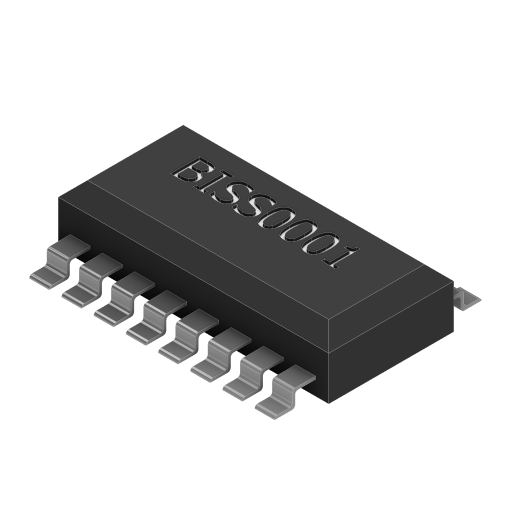
# Autodesk Inventor part: BISS0001 Chip
Saved by Autodesk Inventor 2024 (Build 280153000, 153)
## iProperties
Created: 2024-09-23
Part Number: BISS0001 Chip
Material: Generic
Document SubType Name: Modeling
Designer: Laith Al-Sadi
Density: 1 g/cm^3
Appearance: Rubber - Black
Author: Laith Al-Sadi
Autodesk Inventor part; units mm, degrees
ref_plane "YZ Plane" through (0, 0, 0) normal (1, 0, 0) x (0, 1, 0)
ref_plane "XZ Plane" through (0, 0, 0) normal (0, 1, 0) x (-1, 0, 0)
sketch "Sketch1" plane through (0, 0, 0) normal (0, 1, 0) x (-1, 0, 0)
  line L0 (4.62, 2.135) -> (-4.62, 2.135)
  line L1 (-4.62, 2.135) -> (-4.62, -2.135)
  line L2 (-4.62, -2.135) -> (4.62, -2.135)
  line L3 (4.62, -2.135) -> (4.62, 2.135)
  line L4 (4.62, 2.135) -> (-4.62, -2.135) construction
  line L5 (-4.62, 2.135) -> (4.62, -2.135) construction
  point P0 (0, 0)
  dimension "d0" = 9.24
  dimension "d1" = 4.27
  constraints: 12 end point, 2 midpoint, 2 parallel, 1 horizontal, 1 perpendicular
  measures "d0" distance of L1.end L2.end
  measures "d1" distance of L2.end L0.start
extrude "Extrusion1" add sketch "Sketch1" along normal blind 2
chamfer "Chamfer1" distance 0.5 angle 45 4 edges at (0, 2, 2.135) (-4.62, 2, 0) (0, 2, -2.135) (4.62, 2, 0)
sketch "Sketch2" plane through (0, 2, 0) normal (0, 1, 0) x (1, 0, 0)
  line L0 (-3, 1) -> (3, 1) construction
  line L1 (3, 1) -> (3, -1) construction
  line L2 (3, -1) -> (-3, -1) construction
  line L3 (-3, -1) -> (-3, 1) construction
  spline S0 degree 2 poles (-2.2204, 0.2869) (-2.2204, 0.2123) (-2.2771, 0.0981) (-2.3241, 0.0608) knots 0 0 0 1 2 2 2
  spline S1 degree 2 poles (-2.3241, 0.0608) (-2.3809, 0.017) (-2.5097, -0.0203) (-2.6118, -0.0203) knots 0 0 0 1 2 2 2
  line L4 (-2.6118, -0.0203) -> (-2.8987, -0.0203)
  line L5 (-2.8987, -0.0203) -> (-2.8987, 0.9797)
  line L6 (-2.8987, 0.9797) -> (-2.6337, 0.9797)
  spline S2 degree 2 poles (-2.6337, 0.9797) (-2.5267, 0.9797) (-2.4198, 0.966) (-2.3712, 0.9392) knots 0 0 0 1 2 2 2
  spline S3 degree 2 poles (-2.3712, 0.9392) (-2.3169, 0.9109) (-2.2674, 0.8177) (-2.2674, 0.7545) knots 0 0 0 1 2 2 2
  spline S4 degree 2 poles (-2.2674, 0.7545) (-2.2674, 0.684) (-2.342, 0.5721) (-2.4076, 0.5405) knots 0 0 0 1 2 2 2
  line L7 (-2.4076, 0.5405) -> (-2.4076, 0.5357)
  spline S5 degree 2 poles (-2.4076, 0.5357) (-2.3185, 0.5113) (-2.2204, 0.3825) (-2.2204, 0.2869) knots 0 0 0 1 2 2 2
  spline S6 degree 2 poles (-2.359, 0.2812) (-2.359, 0.3379) (-2.3914, 0.4109) (-2.44, 0.4368) knots 0 0 0 1 2 2 2
  spline S7 degree 2 poles (-2.44, 0.4368) (-2.4716, 0.453) (-2.5462, 0.4627) (-2.6151, 0.4627) knots 0 0 0 1 2 2 2
  line L8 (-2.6151, 0.4627) -> (-2.7658, 0.4627)
  line L9 (-2.7658, 0.4627) -> (-2.7658, 0.0932)
  line L10 (-2.7658, 0.0932) -> (-2.658, 0.0932)
  spline S8 degree 2 poles (-2.658, 0.0932) (-2.5705, 0.0932) (-2.47, 0.1094) (-2.4311, 0.1353) knots 0 0 0 1 2 2 2
  spline S9 degree 2 poles (-2.4311, 0.1353) (-2.3938, 0.1621) (-2.359, 0.2285) (-2.359, 0.2812) knots 0 0 0 1 2 2 2
  spline S10 degree 2 poles (-2.406, 0.7358) (-2.406, 0.7715) (-2.4303, 0.825) (-2.4571, 0.8404) knots 0 0 0 1 2 2 2
  spline S11 degree 2 poles (-2.4571, 0.8404) (-2.4895, 0.8582) (-2.5681, 0.8663) (-2.6386, 0.8663) knots 0 0 0 1 2 2 2
  line L11 (-2.6386, 0.8663) -> (-2.7658, 0.8663)
  line L12 (-2.7658, 0.8663) -> (-2.7658, 0.5737)
  line L13 (-2.7658, 0.5737) -> (-2.6151, 0.5737)
  spline S12 degree 2 poles (-2.6151, 0.5737) (-2.5527, 0.5737) (-2.4935, 0.5867) (-2.4619, 0.607) knots 0 0 0 1 2 2 2
  spline S13 degree 2 poles (-2.4619, 0.607) (-2.4311, 0.6264) (-2.406, 0.6888) (-2.406, 0.7358) knots 0 0 0 1 2 2 2
  line L14 (-1.7399, -0.0203) -> (-2.1272, -0.0203)
  line L15 (-2.1272, -0.0203) -> (-2.1272, 0.0818)
  line L16 (-2.1272, 0.0818) -> (-2, 0.0818)
  line L17 (-2, 0.0818) -> (-2, 0.8776)
  line L18 (-2, 0.8776) -> (-2.1272, 0.8776)
  line L19 (-2.1272, 0.8776) -> (-2.1272, 0.9797)
  line L20 (-2.1272, 0.9797) -> (-1.7399, 0.9797)
  line L21 (-1.7399, 0.9797) -> (-1.7399, 0.8776)
  line L22 (-1.7399, 0.8776) -> (-1.8671, 0.8776)
  line L23 (-1.8671, 0.8776) -> (-1.8671, 0.0818)
  line L24 (-1.8671, 0.0818) -> (-1.7399, 0.0818)
  line L25 (-1.7399, 0.0818) -> (-1.7399, -0.0203)
  spline S14 degree 2 poles (-1.2966, -0.0381) (-1.4052, -0.0381) (-1.5575, 0.0073) (-1.6248, 0.0397) knots 0 0 0 1 2 2 2
  line L26 (-1.6248, 0.0397) -> (-1.6248, 0.2066)
  line L27 (-1.6248, 0.2066) -> (-1.6151, 0.2066)
  spline S15 degree 2 poles (-1.6151, 0.2066) (-1.5494, 0.1451) (-1.3833, 0.077) (-1.3063, 0.077) knots 0 0 0 1 2 2 2
  spline S16 degree 2 poles (-1.3063, 0.077) (-1.1961, 0.077) (-1.0835, 0.1686) (-1.0835, 0.2439) knots 0 0 0 1 2 2 2
  spline S17 degree 2 poles (-1.0835, 0.2439) (-1.0835, 0.3039) (-1.1426, 0.3784) (-1.2066, 0.3971) knots 0 0 0 1 2 2 2
  spline S18 degree 2 poles (-1.2066, 0.3971) (-1.2528, 0.41) (-1.3298, 0.4279) (-1.3874, 0.4425) knots 0 0 0 1 2 2 2
  spline S19 degree 2 poles (-1.3874, 0.4425) (-1.4392, 0.4562) (-1.5211, 0.4976) (-1.5527, 0.5308) knots 0 0 0 1 2 2 2
  spline S20 degree 2 poles (-1.5527, 0.5308) (-1.5835, 0.564) (-1.6175, 0.6532) (-1.6175, 0.7115) knots 0 0 0 1 2 2 2
  spline S21 degree 2 poles (-1.6175, 0.7115) (-1.6175, 0.8331) (-1.4279, 0.9976) (-1.2812, 0.9976) knots 0 0 0 1 2 2 2
  spline S22 degree 2 poles (-1.2812, 0.9976) (-1.1969, 0.9976) (-1.0478, 0.9643) (-0.9838, 0.9327) knots 0 0 0 1 2 2 2
  line L28 (-0.9838, 0.9327) -> (-0.9838, 0.7739)
  line L29 (-0.9838, 0.7739) -> (-0.9935, 0.7739)
  spline S23 degree 2 poles (-0.9935, 0.7739) (-1.0413, 0.8177) (-1.1904, 0.8825) (-1.2723, 0.8825) knots 0 0 0 1 2 2 2
  spline S24 degree 2 poles (-1.2723, 0.8825) (-1.3647, 0.8825) (-1.4789, 0.7958) (-1.4789, 0.7253) knots 0 0 0 1 2 2 2
  spline S25 degree 2 poles (-1.4789, 0.7253) (-1.4789, 0.6621) (-1.4117, 0.5867) (-1.3485, 0.5697) knots 0 0 0 1 2 2 2
  spline S26 degree 2 poles (-1.3485, 0.5697) (-1.3063, 0.5583) (-1.184, 0.5292) (-1.1434, 0.517) knots 0 0 0 1 2 2 2
  spline S27 degree 2 poles (-1.1434, 0.517) (-1.0405, 0.4854) (-0.9449, 0.3582) (-0.9449, 0.265) knots 0 0 0 1 2 2 2
  spline S28 degree 2 poles (-0.9449, 0.265) (-0.9449, 0.2058) (-0.9927, 0.0924) (-1.0357, 0.0527) knots 0 0 0 1 2 2 2
  spline S29 degree 2 poles (-1.0357, 0.0527) (-1.0835, 0.0089) (-1.205, -0.0381) (-1.2966, -0.0381) knots 0 0 0 1 2 2 2
  spline S30 degree 2 poles (-0.5308, -0.0381) (-0.6394, -0.0381) (-0.7917, 0.0073) (-0.859, 0.0397) knots 0 0 0 1 2 2 2
  line L30 (-0.859, 0.0397) -> (-0.859, 0.2066)
  line L31 (-0.859, 0.2066) -> (-0.8493, 0.2066)
  spline S31 degree 2 poles (-0.8493, 0.2066) (-0.7836, 0.1451) (-0.6175, 0.077) (-0.5405, 0.077) knots 0 0 0 1 2 2 2
  spline S32 degree 2 poles (-0.5405, 0.077) (-0.4303, 0.077) (-0.3177, 0.1686) (-0.3177, 0.2439) knots 0 0 0 1 2 2 2
  spline S33 degree 2 poles (-0.3177, 0.2439) (-0.3177, 0.3039) (-0.3768, 0.3784) (-0.4408, 0.3971) knots 0 0 0 1 2 2 2
  spline S34 degree 2 poles (-0.4408, 0.3971) (-0.487, 0.41) (-0.564, 0.4279) (-0.6216, 0.4425) knots 0 0 0 1 2 2 2
  spline S35 degree 2 poles (-0.6216, 0.4425) (-0.6734, 0.4562) (-0.7553, 0.4976) (-0.7869, 0.5308) knots 0 0 0 1 2 2 2
  spline S36 degree 2 poles (-0.7869, 0.5308) (-0.8177, 0.564) (-0.8517, 0.6532) (-0.8517, 0.7115) knots 0 0 0 1 2 2 2
  spline S37 degree 2 poles (-0.8517, 0.7115) (-0.8517, 0.8331) (-0.6621, 0.9976) (-0.5154, 0.9976) knots 0 0 0 1 2 2 2
  spline S38 degree 2 poles (-0.5154, 0.9976) (-0.4311, 0.9976) (-0.282, 0.9643) (-0.218, 0.9327) knots 0 0 0 1 2 2 2
  line L32 (-0.218, 0.9327) -> (-0.218, 0.7739)
  line L33 (-0.218, 0.7739) -> (-0.2277, 0.7739)
  spline S39 degree 2 poles (-0.2277, 0.7739) (-0.2755, 0.8177) (-0.4246, 0.8825) (-0.5065, 0.8825) knots 0 0 0 1 2 2 2
  spline S40 degree 2 poles (-0.5065, 0.8825) (-0.5989, 0.8825) (-0.7131, 0.7958) (-0.7131, 0.7253) knots 0 0 0 1 2 2 2
  spline S41 degree 2 poles (-0.7131, 0.7253) (-0.7131, 0.6621) (-0.6459, 0.5867) (-0.5827, 0.5697) knots 0 0 0 1 2 2 2
  spline S42 degree 2 poles (-0.5827, 0.5697) (-0.5405, 0.5583) (-0.4182, 0.5292) (-0.3776, 0.517) knots 0 0 0 1 2 2 2
  spline S43 degree 2 poles (-0.3776, 0.517) (-0.2747, 0.4854) (-0.1791, 0.3582) (-0.1791, 0.265) knots 0 0 0 1 2 2 2
  spline S44 degree 2 poles (-0.1791, 0.265) (-0.1791, 0.2058) (-0.2269, 0.0924) (-0.2699, 0.0527) knots 0 0 0 1 2 2 2
  spline S45 degree 2 poles (-0.2699, 0.0527) (-0.3177, 0.0089) (-0.4392, -0.0381) (-0.5308, -0.0381) knots 0 0 0 1 2 2 2
  spline S46 degree 2 poles (0.5502, 0.4797) (0.5502, 0.2107) (0.3938, -0.0413) (0.231, -0.0413) knots 0 0 0 1 2 2 2
  spline S47 degree 2 poles (0.231, -0.0413) (0.0656, -0.0413) (-0.0891, 0.2156) (-0.0891, 0.4789) knots 0 0 0 1 2 2 2
  spline S48 degree 2 poles (-0.0891, 0.4789) (-0.0891, 0.7496) (0.0673, 1) (0.231, 1) knots 0 0 0 1 2 2 2
  spline S49 degree 2 poles (0.231, 1) (0.3955, 1) (0.5502, 0.7407) (0.5502, 0.4797) knots 0 0 0 1 2 2 2
  spline S50 degree 2 poles (0.3784, 0.175) (0.3979, 0.2245) (0.4141, 0.3768) (0.4141, 0.4797) knots 0 0 0 1 2 2 2
  spline S51 degree 2 poles (0.4141, 0.4797) (0.4141, 0.5827) (0.3979, 0.7342) (0.3776, 0.7853) knots 0 0 0 1 2 2 2
  spline S52 degree 2 poles (0.3776, 0.7853) (0.3574, 0.8363) (0.2869, 0.889) (0.231, 0.889) knots 0 0 0 1 2 2 2
  spline S53 degree 2 poles (0.231, 0.889) (0.175, 0.889) (0.1029, 0.8363) (0.0818, 0.7836) knots 0 0 0 1 2 2 2
  spline S54 degree 2 poles (0.0818, 0.7836) (0.0616, 0.7326) (0.047, 0.577) (0.047, 0.4789) knots 0 0 0 1 2 2 2
  spline S55 degree 2 poles (0.047, 0.4789) (0.047, 0.3736) (0.06, 0.2326) (0.081, 0.1775) knots 0 0 0 1 2 2 2
  spline S56 degree 2 poles (0.081, 0.1775) (0.1005, 0.1256) (0.1726, 0.0697) (0.231, 0.0697) knots 0 0 0 1 2 2 2
  spline S57 degree 2 poles (0.231, 0.0697) (0.2861, 0.0697) (0.3582, 0.1224) (0.3784, 0.175) knots 0 0 0 1 2 2 2
  spline S58 degree 2 poles (1.3006, 0.4797) (1.3006, 0.2107) (1.1442, -0.0413) (0.9814, -0.0413) knots 0 0 0 1 2 2 2
  spline S59 degree 2 poles (0.9814, -0.0413) (0.816, -0.0413) (0.6613, 0.2156) (0.6613, 0.4789) knots 0 0 0 1 2 2 2
  spline S60 degree 2 poles (0.6613, 0.4789) (0.6613, 0.7496) (0.8177, 1) (0.9814, 1) knots 0 0 0 1 2 2 2
  spline S61 degree 2 poles (0.9814, 1) (1.1459, 1) (1.3006, 0.7407) (1.3006, 0.4797) knots 0 0 0 1 2 2 2
  spline S62 degree 2 poles (1.1288, 0.175) (1.1483, 0.2245) (1.1645, 0.3768) (1.1645, 0.4797) knots 0 0 0 1 2 2 2
  spline S63 degree 2 poles (1.1645, 0.4797) (1.1645, 0.5827) (1.1483, 0.7342) (1.128, 0.7853) knots 0 0 0 1 2 2 2
  spline S64 degree 2 poles (1.128, 0.7853) (1.1078, 0.8363) (1.0373, 0.889) (0.9814, 0.889) knots 0 0 0 1 2 2 2
  spline S65 degree 2 poles (0.9814, 0.889) (0.9254, 0.889) (0.8533, 0.8363) (0.8323, 0.7836) knots 0 0 0 1 2 2 2
  spline S66 degree 2 poles (0.8323, 0.7836) (0.812, 0.7326) (0.7974, 0.577) (0.7974, 0.4789) knots 0 0 0 1 2 2 2
  spline S67 degree 2 poles (0.7974, 0.4789) (0.7974, 0.3736) (0.8104, 0.2326) (0.8314, 0.1775) knots 0 0 0 1 2 2 2
  spline S68 degree 2 poles (0.8314, 0.1775) (0.8509, 0.1256) (0.923, 0.0697) (0.9814, 0.0697) knots 0 0 0 1 2 2 2
  spline S69 degree 2 poles (0.9814, 0.0697) (1.0365, 0.0697) (1.1086, 0.1224) (1.1288, 0.175) knots 0 0 0 1 2 2 2
  spline S70 degree 2 poles (2.0511, 0.4797) (2.0511, 0.2107) (1.8947, -0.0413) (1.7318, -0.0413) knots 0 0 0 1 2 2 2
  spline S71 degree 2 poles (1.7318, -0.0413) (1.5665, -0.0413) (1.4117, 0.2156) (1.4117, 0.4789) knots 0 0 0 1 2 2 2
  spline S72 degree 2 poles (1.4117, 0.4789) (1.4117, 0.7496) (1.5681, 1) (1.7318, 1) knots 0 0 0 1 2 2 2
  spline S73 degree 2 poles (1.7318, 1) (1.8963, 1) (2.0511, 0.7407) (2.0511, 0.4797) knots 0 0 0 1 2 2 2
  spline S74 degree 2 poles (1.8793, 0.175) (1.8987, 0.2245) (1.9149, 0.3768) (1.9149, 0.4797) knots 0 0 0 1 2 2 2
  spline S75 degree 2 poles (1.9149, 0.4797) (1.9149, 0.5827) (1.8987, 0.7342) (1.8784, 0.7853) knots 0 0 0 1 2 2 2
  spline S76 degree 2 poles (1.8784, 0.7853) (1.8582, 0.8363) (1.7877, 0.889) (1.7318, 0.889) knots 0 0 0 1 2 2 2
  spline S77 degree 2 poles (1.7318, 0.889) (1.6759, 0.889) (1.6037, 0.8363) (1.5827, 0.7836) knots 0 0 0 1 2 2 2
  spline S78 degree 2 poles (1.5827, 0.7836) (1.5624, 0.7326) (1.5478, 0.577) (1.5478, 0.4789) knots 0 0 0 1 2 2 2
  spline S79 degree 2 poles (1.5478, 0.4789) (1.5478, 0.3736) (1.5608, 0.2326) (1.5818, 0.1775) knots 0 0 0 1 2 2 2
  spline S80 degree 2 poles (1.5818, 0.1775) (1.6013, 0.1256) (1.6734, 0.0697) (1.7318, 0.0697) knots 0 0 0 1 2 2 2
  spline S81 degree 2 poles (1.7318, 0.0697) (1.7869, 0.0697) (1.859, 0.1224) (1.8793, 0.175) knots 0 0 0 1 2 2 2
  line L34 (2.7455, -0.0203) -> (2.2577, -0.0203)
  line L35 (2.2577, -0.0203) -> (2.2577, 0.0818)
  line L36 (2.2577, 0.0818) -> (2.4392, 0.0818)
  line L37 (2.4392, 0.0818) -> (2.4392, 0.752)
  line L38 (2.4392, 0.752) -> (2.2577, 0.752)
  line L39 (2.2577, 0.752) -> (2.2577, 0.8436)
  spline S82 degree 2 poles (2.2577, 0.8436) (2.3606, 0.8436) (2.4579, 0.9019) (2.4643, 0.983) knots 0 0 0 1 2 2 2
  line L40 (2.4643, 0.983) -> (2.5681, 0.983)
  line L41 (2.5681, 0.983) -> (2.5681, 0.0818)
  line L42 (2.5681, 0.0818) -> (2.7455, 0.0818)
  line L43 (2.7455, 0.0818) -> (2.7455, -0.0203)
  point P0 (0, 0)
  point P1 (3, 0)
  point P2 (0, 1)
  dimension "d7" = 6
  dimension "d8" = 2
  constraints: 2 midpoint, 1 horizontal, 1 horizontal alignment, 1 vertical alignment, 2 other
  measures "d7" distance of L0.start L0.end
  measures "d8" distance of L0.end L1.end
extrude "Extrusion2" cut sketch "Sketch2" against normal blind 0.1
ref_plane "Work Plane1" through (4.17, 0, 2.135) normal (1, 0, 0) x (0, 0, -1)
sketch "Sketch4" plane through (4.17, 0, 2.135) normal (1, 0, 0) x (0, 0, -1)
  line L0 (0, 0) -> (0, 1.5) projected
  line L1 (0, 0.5) -> (-0.6, 0.5)
  line L2 (-0.7, 0.4) -> (-0.7, 0.1)
  line L3 (-0.8, 0) -> (-1.4, 0)
  line L4 (0, 0) -> (4.27, 0) projected
  line L5 (0, 0.6) -> (-0.7, 0.6)
  line L6 (-0.8, 0.5) -> (-0.8, 0.2)
  line L7 (-0.9, 0.1) -> (-1.3, 0.1)
  line L8 (-1.4, 0) -> (-1.4, 0)
  line L9 (0, 0.6) -> (0, 0.5)
  arc A0 (-0.6, 0.5) -> (-0.7, 0.4) centre (-0.6, 0.4) ccw
  arc A1 (-0.7, 0.6) -> (-0.8, 0.5) centre (-0.7, 0.5) ccw
  arc A2 (-0.9, 0.1) -> (-0.8, 0.2) centre (-0.9, 0.2) ccw
  arc A3 (-0.8, 0) -> (-0.7, 0.1) centre (-0.8, 0.1) ccw
  arc A4 (-1.3, 0.1) -> (-1.4, 0) centre (-1.3, 0) ccw
  point P0 (2.135, 0)
  point P1 (-0.7, 0.5)
  point P2 (-0.7, 0)
  point P3 (-1.4, 0)
  point P4 (0, 0.6)
  dimension "d12" = 0.7
  dimension "d13" = 0.5
  dimension "d14" = 0.5
  dimension "d15" = 0.7
  dimension "d16" = 0.1
  dimension "d17" = 0.1
  constraints: 16 end point, 10 point on circle, 10 tangent, 5 centre point, 5 perpendicular, 5 point on line, 4 equal radius, 1 collinear, 1 horizontal, 1 vertical, 2 other
  measures "d12" distance of L1.start point (-0.7, 0.5)
  measures "d13" distance of point (-0.7, 0.5) point (-0.7, 0)
  measures "d14" distance between parallel lines of L4 L1
  measures "d15" distance of point (-0.7, 0) L3.end
  measures "d16" distance between parallel lines of L1 L5
  measures "d17" radius of A0
extrude "Extrusion3" add sketch "Sketch4" against normal blind 0.68
pattern_linear "Rectangular Pattern1" count 8 spacing 1.1 along (-1, 0, 0) of "Extrusion3"
mirror "Mirror1" about plane through (0, 0, 0) normal (0, 0, 1) of "Extrusion3", "Rectangular Pattern1"
body "Solid1"
